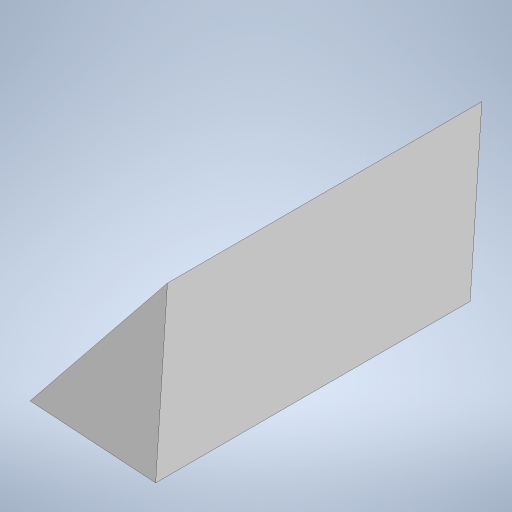
# Autodesk Inventor part: prod
Saved by Autodesk Inventor 2023 (Build 270158000, 158)
## iProperties
Created: 2024-04-25
Part Number: prod
Material: Ogólny
Document SubType Name: Modeling
Designer: Kamil
Density: 1 g/cm^3
Appearance: Domyślna
Author: Kamil
Autodesk Inventor part; units mm, degrees
ref_plane "YZ Plane" through (0, 0, 0) normal (1, 0, 0) x (0, 1, 0)
ref_plane "XZ Plane" through (0, 0, 0) normal (0, 1, 0) x (-1, 0, 0)
ref_plane "XY Plane" through (0, 0, 0) normal (0, 0, 1) x (1, 0, 0)
sketch "Szkic1" plane through (0, 0, 0) normal (0, 0, 1) x (1, 0, 0)
  line L0 (33, 9) -> (29.265, -47.8775)
  line L1 (29.265, -47.8775) -> (-10.649, -45.2564)
  line L2 (-10.649, -45.2564) -> (33, 9)
  point P0 (0, 0)
  dimension "d0" = 40
  dimension "d1" = 57
  constraints: 6 end point, 1 perpendicular
  measures "d0" distance of L0.end L1.end
  measures "d1" distance of L0.start L0.end
extrude "Wyciągnięcie proste1" add sketch "Szkic1" along normal blind 100
